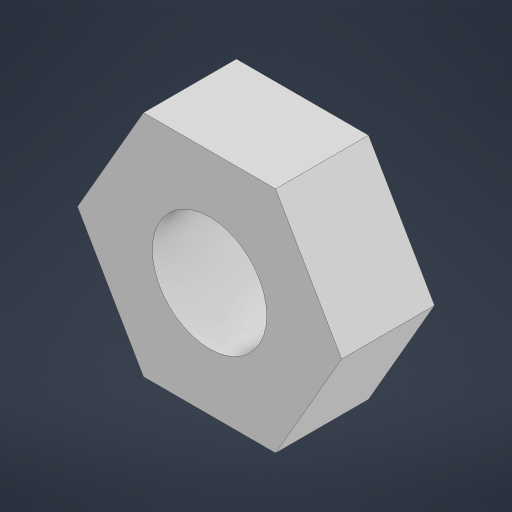
# Autodesk Inventor part: m1.6_nut
Saved by Autodesk Inventor 2023.5 (Build 275446000, 446)
## iProperties
Created: 2025-01-11
Part Number: m1.6_nut
Material: 一般
Document SubType Name: Modeling
Designer: IshiiLabHonda
Density: 1 g/cm^3
Appearance: 既定
Author: IshiiLabHonda
Autodesk Inventor part; units mm, degrees
ref_plane "YZ Plane" through (0, 0, 0) normal (1, 0, 0) x (0, 1, 0)
ref_plane "XZ Plane" through (0, 0, 0) normal (0, 1, 0) x (-1, 0, 0)
ref_plane "XY Plane" through (0, 0, 0) normal (0, 0, 1) x (1, 0, 0)
sketch "スケッチ1" plane through (0, 0, 0) normal (0, 0, 1) x (1, 0, 0)
  line L0 (0.9238, 1.6) -> (1.8475, 0)
  line L1 (1.8475, 0) -> (0.9238, -1.6)
  line L2 (0.9238, -1.6) -> (-0.9238, -1.6)
  line L3 (-0.9238, -1.6) -> (-1.8475, 0)
  line L4 (-1.8475, 0) -> (-0.9238, 1.6)
  line L5 (-0.9238, 1.6) -> (0.9238, 1.6)
  circle A0 centre (0, 0) radius 0.8
  dimension "d0" = 1.6
  dimension "d1" = 3.2
  constraints: 12 end point, 2 coincident, 1 centre point, 1 horizontal, 13 other
  measures "d0" diameter of A0
  measures "d1" distance between parallel lines of L2 L5
extrude "押し出し1" add sketch "スケッチ1" along normal blind 1.3
